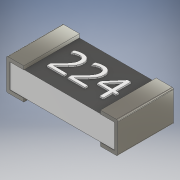
# Autodesk Inventor part: 21-1001
Saved by Autodesk Inventor 2018 (Build 220112000, 112)
## iProperties
Created: 2019-09-21
Part Number: 21-1001
Material: Copper
Document SubType Name: Modeling
Designer: Bradley
Density: 8.94 g/cm^3
Appearance: Smooth - White
Author: Bradley
Autodesk Inventor part; units mm, degrees
ref_plane "YZ Plane" through (0, 0, 0) normal (1, 0, 0) x (0, 1, 0)
ref_plane "XZ Plane" through (0, 0, 0) normal (0, 1, 0) x (-1, 0, 0)
ref_plane "XY Plane" through (0, 0, 0) normal (0, 0, 1) x (1, 0, 0)
sketch "Sketch1" plane through (0, 0, 0) normal (0, 1, 0) x (-1, 0, 0)
  line L0 (0.75, 0.175) -> (-0.75, 0.175)
  line L1 (-0.75, 0.175) -> (-0.75, -0.175)
  line L2 (-0.75, -0.175) -> (0.75, -0.175)
  line L3 (0.75, -0.175) -> (0.75, 0.175)
  line L4 (0.55, 0.175) -> (0.55, 0.225)
  line L5 (0.55, 0.225) -> (0.8, 0.225)
  line L6 (0.8, 0.225) -> (0.8, -0.225)
  line L7 (0.8, -0.225) -> (0.55, -0.225)
  line L8 (0.55, -0.225) -> (0.55, -0.175)
  line L9 (-0.55, 0.175) -> (-0.55, 0.225)
  line L10 (-0.55, 0.225) -> (-0.8, 0.225)
  line L11 (-0.8, 0.225) -> (-0.8, -0.225)
  line L12 (-0.8, -0.225) -> (-0.55, -0.225)
  line L13 (-0.55, -0.175) -> (-0.55, -0.225)
  line L14 (0.55, 0.175) -> (-0.55, 0.175)
  point P0 (0, 0)
  point P1 (0, 0.175)
  point P2 (0.75, 0)
  dimension "d0" = 1.6
  dimension "d1" = 0.05
  dimension "d2" = 0.05
  dimension "d3" = 0.45
  dimension "d4" = 0.25
  constraints: 30 end point, 12 point on line, 7 perpendicular, 3 collinear, 3 midpoint, 2 parallel, 1 horizontal, 1 horizontal alignment, 1 vertical, 1 vertical alignment
  measures "d0" distance between parallel lines of L11 L6
  measures "d1" distance of L7.end L8.end
  measures "d2" distance between parallel lines of L6 L3
  measures "d3" distance of L5.end L6.end
  measures "d4" distance of L6.end L7.end
extrude "Extrusion1" add sketch "Sketch1" along normal mid plane 0.8 contours L0 L4 L5 L6 L7 L8 L2 L3 | L0 L1 L2 L13 L12 L11 L10 L9
extrude "Extrusion2" add sketch "Sketch1" along normal mid plane 0.79 contours L3 L2 L1 L0
sketch "Sketch2" plane through (-0.55, -0.395, 0.175) normal (0, 0, 1) x (1, 0, 0)
  line L0 (0, 0) -> (0, 0.79) projected
  line L1 (1.1, 0) -> (0, 0) projected
  line L2 (1.1, 0) -> (1.1, 0.79) projected
  line L3 (0, 0.79) -> (1.1, 0.79) projected
  line L4 (0, 0.395) -> (1.1, 0.395) construction
  line L5 (0.3756, 0.195) -> (0.1289, 0.195)
  line L6 (0.1289, 0.195) -> (0.1289, 0.2517)
  spline S0 degree 2 poles (0.1289, 0.2517) (0.1555, 0.2767) (0.2028, 0.323) (0.2255, 0.348) knots 0 0 0 1 2 2 2
  spline S1 degree 2 poles (0.2255, 0.348) (0.2712, 0.3982) (0.3046, 0.4585) (0.3046, 0.4906) knots 0 0 0 1 2 2 2
  spline S2 degree 2 poles (0.3046, 0.4906) (0.3046, 0.5075) (0.2942, 0.5328) (0.2848, 0.5409) knots 0 0 0 1 2 2 2
  spline S3 degree 2 poles (0.2848, 0.5409) (0.2754, 0.549) (0.2508, 0.5571) (0.2359, 0.5571) knots 0 0 0 1 2 2 2
  spline S4 degree 2 poles (0.2359, 0.5571) (0.2216, 0.5571) (0.1925, 0.5499) (0.1792, 0.5444) knots 0 0 0 1 2 2 2
  spline S5 degree 2 poles (0.1792, 0.5444) (0.1678, 0.5399) (0.1468, 0.5269) (0.1403, 0.5224) knots 0 0 0 1 2 2 2
  line L7 (0.1403, 0.5224) -> (0.1374, 0.5224)
  line L8 (0.1374, 0.5224) -> (0.1374, 0.5794)
  spline S6 degree 2 poles (0.1374, 0.5794) (0.1539, 0.5875) (0.2132, 0.6034) (0.2398, 0.6034) knots 0 0 0 1 2 2 2
  spline S7 degree 2 poles (0.2398, 0.6034) (0.2959, 0.6034) (0.3591, 0.5441) (0.3591, 0.4935) knots 0 0 0 1 2 2 2
  spline S8 degree 2 poles (0.3591, 0.4935) (0.3591, 0.4699) (0.3481, 0.4303) (0.3383, 0.4135) knots 0 0 0 1 2 2 2
  spline S9 degree 2 poles (0.3383, 0.4135) (0.3286, 0.396) (0.3004, 0.3616) (0.2848, 0.3451) knots 0 0 0 1 2 2 2
  spline S10 degree 2 poles (0.2848, 0.3451) (0.2596, 0.3175) (0.1976, 0.2585) (0.1792, 0.2414) knots 0 0 0 1 2 2 2
  line L9 (0.1792, 0.2414) -> (0.3756, 0.2414)
  line L10 (0.3756, 0.2414) -> (0.3756, 0.195)
  line L11 (0.6758, 0.195) -> (0.4291, 0.195)
  line L12 (0.4291, 0.195) -> (0.4291, 0.2517)
  spline S11 degree 2 poles (0.4291, 0.2517) (0.4557, 0.2767) (0.503, 0.323) (0.5257, 0.348) knots 0 0 0 1 2 2 2
  spline S12 degree 2 poles (0.5257, 0.348) (0.5714, 0.3982) (0.6048, 0.4585) (0.6048, 0.4906) knots 0 0 0 1 2 2 2
  spline S13 degree 2 poles (0.6048, 0.4906) (0.6048, 0.5075) (0.5944, 0.5328) (0.585, 0.5409) knots 0 0 0 1 2 2 2
  spline S14 degree 2 poles (0.585, 0.5409) (0.5756, 0.549) (0.551, 0.5571) (0.5361, 0.5571) knots 0 0 0 1 2 2 2
  spline S15 degree 2 poles (0.5361, 0.5571) (0.5218, 0.5571) (0.4926, 0.5499) (0.4793, 0.5444) knots 0 0 0 1 2 2 2
  spline S16 degree 2 poles (0.4793, 0.5444) (0.468, 0.5399) (0.4469, 0.5269) (0.4404, 0.5224) knots 0 0 0 1 2 2 2
  line L13 (0.4404, 0.5224) -> (0.4375, 0.5224)
  line L14 (0.4375, 0.5224) -> (0.4375, 0.5794)
  spline S17 degree 2 poles (0.4375, 0.5794) (0.4541, 0.5875) (0.5134, 0.6034) (0.54, 0.6034) knots 0 0 0 1 2 2 2
  spline S18 degree 2 poles (0.54, 0.6034) (0.596, 0.6034) (0.6592, 0.5441) (0.6592, 0.4935) knots 0 0 0 1 2 2 2
  spline S19 degree 2 poles (0.6592, 0.4935) (0.6592, 0.4699) (0.6482, 0.4303) (0.6385, 0.4135) knots 0 0 0 1 2 2 2
  spline S20 degree 2 poles (0.6385, 0.4135) (0.6288, 0.396) (0.6006, 0.3616) (0.585, 0.3451) knots 0 0 0 1 2 2 2
  spline S21 degree 2 poles (0.585, 0.3451) (0.5597, 0.3175) (0.4978, 0.2585) (0.4793, 0.2414) knots 0 0 0 1 2 2 2
  line L15 (0.4793, 0.2414) -> (0.6758, 0.2414)
  line L16 (0.6758, 0.2414) -> (0.6758, 0.195)
  line L17 (0.9866, 0.3324) -> (0.939, 0.3324)
  line L18 (0.939, 0.3324) -> (0.939, 0.195)
  line L19 (0.939, 0.195) -> (0.8874, 0.195)
  line L20 (0.8874, 0.195) -> (0.8874, 0.3324)
  line L21 (0.8874, 0.3324) -> (0.7108, 0.3324)
  line L22 (0.7108, 0.3324) -> (0.7108, 0.3888)
  line L23 (0.7108, 0.3888) -> (0.8897, 0.595)
  line L24 (0.8897, 0.595) -> (0.939, 0.595)
  line L25 (0.939, 0.595) -> (0.939, 0.3756)
  line L26 (0.939, 0.3756) -> (0.9866, 0.3756)
  line L27 (0.9866, 0.3756) -> (0.9866, 0.3324)
  line L28 (0.8874, 0.3756) -> (0.8874, 0.5318)
  line L29 (0.8874, 0.5318) -> (0.7529, 0.3756)
  line L30 (0.7529, 0.3756) -> (0.8874, 0.3756)
  point P0 (0.55, 0.395)
  constraints: 2 end point, 2 midpoint, 1 horizontal
extrude "Extrusion3" add sketch "Sketch2" along normal blind 0.02 contours L5 L6 S0 S1 S2 S3 S4 S5 L7 L8 S6 S7 S8 S9 S10 L9 L10 | L11 L12 S11 S12 S13 S14 S15 S16 L13 L14 S17 S18 S19 S20 S21 L15 L16 | L17 L18 L19 L20 L21 L22 L23 L24 L25 L26 L27
fillet "Fillet1" radius 0.02 4 edges at (-0.8, 0, 0.225) (-0.8, 0, -0.225) (0.8, 0, 0.225) (0.8, 0, -0.225)
equation "\"d2\" = d1"
body "Solid1"
